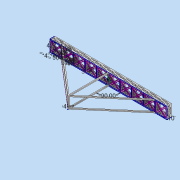
# Autodesk Inventor part: hashi1shado
Saved by Autodesk Inventor 2022 (Build 260153000, 153)
## iProperties
Created: 2024-05-14
Part Number: hashi1shado
Material: 一般
Document SubType Name: Modeling
Designer: ktamu
Density: 1 g/cm^3
Appearance: 既定
Mass: 137.691 g
Surface Area: 1271.48 cm^2
Volume: 137.691 cm^3
Author: ktamu
Autodesk Inventor part; units mm, degrees
ref_plane "YZ Plane" through (0, 0, 0) normal (1, 0, 0) x (0, 1, 0)
ref_plane "XZ Plane" through (0, 0, 0) normal (0, 1, 0) x (-1, 0, 0)
ref_plane "XY Plane" through (0, 0, 0) normal (0, 0, 1) x (1, 0, 0)
sketch "スケッチ2" plane through (0, 0, 0) normal (1, 0, 0) x (0, 1, 0)
  line L0 (25, 10) -> (-25, 10)
  line L1 (-25, 10) -> (-25, -10)
  line L2 (-25, -10) -> (25, -10)
  line L3 (25, -10) -> (25, 10)
  line L4 (25, 10) -> (-25, -10) construction
  line L5 (-25, 10) -> (25, -10) construction
  point P0 (0, 0)
  dimension "d4" = 50
  dimension "d5" = 20
  constraints: 12 end point, 2 midpoint, 2 parallel, 1 horizontal, 1 perpendicular
  measures "d4" distance of L2.end L1.end
  measures "d5" distance of L1.end L0.end
extrude "押し出し2" add sketch "スケッチ2" along normal mid plane 500
sketch "スケッチ3" plane through (-250, -25, 10) normal (0, 0, 1) x (1, 0, 0)
  circle A0 centre (250, 25) radius 5
  dimension "d8" = 10
  constraints: 1 centre point, 1 coincident
  measures "d8" diameter of A0
extrude "押し出し3" add sketch "スケッチ3" along normal blind 2
sketch "SCfront" plane through (-250, -25, 10) normal (0, -1, 0) x (1, 0, 0)
  line L0 (0, -20) -> (500, -20) projected
  line L1 (500, 0) -> (500, -20) projected
  line L2 (500, 0) -> (0, 0) projected
  line L3 (0, -20) -> (0, 0) projected
  line L4 (0, 0) -> (500, 0)
  line L5 (500, 0) -> (500, -20)
  line L6 (500, -20) -> (0, -20)
  line L7 (0, -20) -> (0, 0)
  line L8 (0, 0) -> (500, -20) construction
  line L9 (500, 0) -> (0, -20) construction
  line L10 (0, 0) -> (500, 0) projected
  line L11 (0, -20) -> (500, -20) projected
  line L12 (0, 0) -> (50, 0)
  line L13 (50, 0) -> (50, -20)
  line L14 (50, -20) -> (0, -20)
  line L15 (0, -20) -> (0, 0)
  line L16 (100, 0) -> (100, -20)
  line L17 (150, 0) -> (150, -20)
  line L18 (200, 0) -> (200, -20)
  line L19 (250, 0) -> (250, -20)
  line L20 (450, 0) -> (450, -20)
  line L21 (400, 0) -> (400, -20)
  line L22 (350, 0) -> (350, -20)
  line L23 (300, 0) -> (300, -20)
  line L24 (0, 0) -> (0, -20) projected
  line L25 (0, 0) -> (50, -20)
  line L26 (0, -20) -> (50, 0) construction
  line L27 (50, 0) -> (100, -20)
  line L28 (100, 0) -> (50, -20)
  line L29 (52, -4) -> (98, -4)
  line L30 (98, -4) -> (98, -16)
  line L31 (98, -16) -> (52, -16)
  line L32 (52, -16) -> (52, -4)
  line L33 (75, -10) -> (98, -16) construction
  line L34 (98, -4) -> (52, -16) construction
  line L35 (102, -4) -> (148, -4)
  line L36 (102, -16) -> (102, -4)
  line L37 (148, -16) -> (102, -16)
  line L38 (148, -4) -> (148, -16)
  line L39 (152, -4) -> (198, -4)
  line L40 (152, -16) -> (152, -4)
  line L41 (198, -16) -> (152, -16)
  line L42 (198, -4) -> (198, -16)
  line L43 (202, -4) -> (248, -4)
  line L44 (202, -16) -> (202, -4)
  line L45 (248, -16) -> (202, -16)
  line L46 (248, -4) -> (248, -16)
  line L47 (252, -4) -> (298, -4)
  line L48 (252, -16) -> (252, -4)
  line L49 (298, -16) -> (252, -16)
  line L50 (298, -4) -> (298, -16)
  line L51 (302, -4) -> (348, -4)
  line L52 (302, -16) -> (302, -4)
  line L53 (348, -16) -> (302, -16)
  line L54 (348, -4) -> (348, -16)
  line L55 (352, -4) -> (398, -4)
  line L56 (352, -16) -> (352, -4)
  line L57 (398, -16) -> (352, -16)
  line L58 (398, -4) -> (398, -16)
  line L59 (402, -4) -> (448, -4)
  line L60 (402, -16) -> (402, -4)
  line L61 (448, -16) -> (402, -16)
  line L62 (448, -4) -> (448, -16)
  line L63 (48, -4) -> (48, -16)
  line L64 (48, -4) -> (4, -4)
  line L65 (4, -4) -> (4, -16.3421)
  line L66 (4, -16.3421) -> (48, -16.3421)
  line L67 (48, -16.3421) -> (48, -4)
  line L68 (452, -4) -> (452, -16)
  line L69 (452, -4) -> (496, -4)
  line L70 (496, -4) -> (496, -16.3421)
  line L71 (496, -16.3421) -> (452, -16.3421)
  line L72 (11.4052, -4) -> (48, -14.2649)
  line L73 (4, -6.0772) -> (40.5948, -16.3421)
  line L74 (488.5948, -4) -> (452, -14.2649)
  line L75 (496, -6.0772) -> (459.4052, -16.3421)
  line L76 (52, -4) -> (75, -10)
  line L77 (52, -6.0669) -> (90.0768, -16)
  line L78 (52.5048, -2.0648) -> (52.6652, -2.1066)
  line L79 (59.9232, -4) -> (98, -13.9331)
  line L80 (109.9232, -4) -> (148, -13.9331)
  line L81 (102, -6.0669) -> (140.0768, -16)
  line L82 (159.9232, -4) -> (198, -13.9331)
  line L83 (152, -6.0669) -> (190.0768, -16)
  line L84 (209.9232, -4) -> (248, -13.9331)
  line L85 (202, -6.0669) -> (240.0768, -16)
  line L86 (448, -6.0669) -> (409.9232, -16)
  line L87 (440.0768, -4) -> (402, -13.9331)
  line L88 (390.0768, -4) -> (352, -13.9331)
  line L89 (398, -6.0669) -> (359.9232, -16)
  line L90 (340.0768, -4) -> (302, -13.9331)
  line L91 (348, -6.0669) -> (309.9232, -16)
  line L92 (290.0768, -4) -> (252, -13.9331)
  line L93 (298, -6.0669) -> (259.9232, -16)
  line L94 (0, -10) -> (496, -10) construction
  line L95 (0, -10) -> (496, -10) construction
  line L96 (11.4052, -16) -> (48, -5.7351)
  line L97 (4, -13.9228) -> (39.375, -4)
  line L98 (488.5948, -16) -> (452, -5.7351)
  line L99 (496, -13.9228) -> (459.4052, -3.6579)
  line L100 (52, -13.9331) -> (90.0768, -4)
  line L101 (59.9232, -16) -> (98, -6.0669)
  line L102 (109.9232, -16) -> (148, -6.0669)
  line L103 (102, -13.9331) -> (140.0768, -4)
  line L104 (159.9232, -16) -> (198, -6.0669)
  line L105 (152, -13.9331) -> (190.0768, -4)
  line L106 (209.9232, -16) -> (248, -6.0669)
  line L107 (202, -13.9331) -> (240.0768, -4)
  line L108 (448, -13.9331) -> (409.9232, -4)
  line L109 (440.0768, -16) -> (402, -6.0669)
  line L110 (398, -13.9331) -> (359.9232, -4)
  line L111 (390.0768, -16) -> (352, -6.0669)
  line L112 (348, -13.9331) -> (309.9232, -4)
  line L113 (340.0768, -16) -> (302, -6.0669)
  line L114 (298, -13.9331) -> (259.9232, -4)
  line L115 (290.0768, -16) -> (252, -6.0669)
  line L116 (25.3901, -12.0772) -> (10.1855, -16.3421)
  line L117 (474.6099, -12.0772) -> (489.8145, -16.3421)
  line L118 (150, 0) -> (313.5157, 0) construction
  line L119 (250, 0) -> (250, 173.2051)
  line L120 (250, 0) -> (423.2051, 0) construction
  line L121 (248, -20) -> (248, 0)
  line L122 (248, 0) -> (248, 166.2211)
  line L123 (152, -0.5359) -> (152, -20)
  line L124 (252, -20) -> (252, 0)
  line L125 (148, 0.5359) -> (148, -20)
  line L126 (250, 173.2051) -> (250, 177.2051)
  line L127 (150, 0) -> (152, 3.4641)
  line L128 (248, 166.2211) -> (54.1451, 0)
  line L129 (48, 0) -> (250, 173.2051)
  point P0 (250, -10)
  point P1 (440.0768, -4)
  point P2 (390.0768, -4)
  point P3 (340.0768, -4)
  point P4 (290.0768, -4)
  point P5 (209.9232, -4)
  point P6 (159.9232, -4)
  point P7 (109.9232, -4)
  point P8 (60.1439, -4.0576)
  point P9 (60, -4)
  point P10 (90, -16)
  point P11 (89.8561, -15.9424)
  point P12 (48, -14.2649)
  point P13 (40.5948, -3.6579)
  point P14 (482.0151, -10)
  point P15 (474.6099, -7.9228)
  point P16 (460.625, -4)
  point P17 (467.2046, -10)
  point P18 (432.9232, -10)
  point P19 (425, -12.0669)
  point P20 (425, -7.9331)
  point P21 (417.0768, -10)
  point P22 (382.9232, -10)
  point P23 (375, -12.0669)
  point P24 (375, -7.9331)
  point P25 (367.0768, -10)
  point P26 (332.9232, -10)
  point P27 (325, -12.0669)
  point P28 (325, -7.9331)
  point P29 (317.0768, -10)
  point P30 (282.9232, -10)
  point P31 (275, -12.0669)
  point P32 (275, -7.9331)
  point P33 (267.0768, -10)
  point P34 (232.9232, -10)
  point P35 (225, -7.9331)
  point P36 (225, -12.0669)
  point P37 (217.0768, -10)
  point P38 (182.9232, -10)
  point P39 (175, -7.9331)
  point P40 (175, -12.0669)
  point P41 (167.0768, -10)
  point P42 (132.9232, -10)
  point P43 (125, -7.9331)
  point P44 (125, -12.0669)
  point P45 (117.0768, -10)
  point P46 (67.0768, -10)
  point P47 (59.9232, -16)
  point P48 (75, -12.0669)
  point P49 (75, -7.9331)
  point P50 (82.9232, -10)
  point P51 (25.3901, -7.9228)
  point P52 (32.7954, -10)
  point P53 (48, -5.7351)
  point P54 (11.4052, -16)
  point P55 (17.9849, -10)
  point P56 (4, -13.9228)
  point P57 (148, 0)
  point P58 (54.1451, 0)
  point P59 (48, 0)
  dimension "d12" = 50
  dimension "d15" = 50
  dimension "d20" = 46
  dimension "d21" = 12
  dimension "d24" = 50
  dimension "d29" = 4
  dimension "d30" = 4
  dimension "d33" = 4
  dimension "d37" = 2
  dimension "d40" = 50
  dimension "d96" = 0
  dimension "d97" = 10
  dimension "d105" = 90
  dimension "d116" = 4
  constraints: 246 end point, 73 symmetric about line, 25 point on line, 12 parallel, 10 horizontal, 6 midpoint, 4 perpendicular, 2 equal length, 1 vertical, 87 other
  measures "d12" distance of L13.end L14.end
  measures "d15" distance of L12.end L16.start
  measures "d20" distance of L30.end L31.end
  measures "d21" distance of L29.end L30.end
  measures "d24" distance of L29.start L35.start
  measures "d29" distance between parallel lines of L32 L63
  measures "d30" distance between parallel lines of L65 L3
  measures "d33" distance between parallel lines of L12 L64
  measures "d37" distance between parallel lines of L76 L77
  measures "d40" distance of L79.start L80.start
  measures "d96" distance between parallel lines of L94 L95
  measures "d97" distance between parallel lines of L0 L95
  measures "d105" angle of L120 L119
  measures "d116" distance between parallel lines of L129 L128
extrude "押し出し4" cut sketch "SCfront" against normal through all contours L31 L101 L28 | L28 L101 L77 L27 L31 | L29 L28 L100 L79 L27 | L66 L116 L96 L73 | L101 L31 L32 L100 L77 L28 | L28 L77 L101 | L64 L97 L72 | L29 L100 L28 | L96 L116 L66 L65 L97 L73 | L96 L63 L72 | L72 L97 L64 L63 L96 | L97 L65 L73 | L37 L102 L81 | L80 L102 L38 | L38 L102 L80 L103 L35 | L100 L29 L30 L101 L79 L28 | L28 L79 L100 | L100 L32 L77 | L37 L36 L103 L81 L102 | L103 L80 L35 | L101 L30 L79 | L46 L106 L84 L107 L43 | L47 L114 L92 L115 L48 | L103 L36 L81 | L107 L84 L43 | L46 L84 L106 | L47 L92 L114 | L115 L92 L48 | L45 L106 L85 | L93 L115 L49 | L107 L44 L85 | L85 L106 L45 L44 L107 | L114 L50 L49 L115 L93 | L93 L50 L114 | L39 L105 L82 | L83 L105 L40 | L39 L42 L104 L82 L105 | L105 L83 L104 L41 L40 | L104 L42 L82 | L83 L41 L104 | L51 L112 L90 L113 L52 | L51 L90 L112 | L113 L90 L52 | L112 L54 L53 L113 L91 | L91 L54 L112 | L113 L53 L91 | L55 L110 L88 L111 L56 | L55 L88 L110 | L111 L88 L56 | L110 L58 L57 L111 L89 | L89 L58 L110 | L111 L57 L89 | L59 L108 L87 L109 L60 | L59 L87 L108 | L109 L87 L60 | L108 L62 L61 L109 L86 | L86 L62 L108 | L109 L61 L86 | L69 L99 L74 L98 L68 | L98 L74 L68 | L69 L74 L99 | L98 L117 L71 L75 | L75 L99 L70 L71 L117 L98 | L75 L70 L99
sketch "SCLeft" plane through (-250, 0, 0) normal (-1, 0, 0) x (0, 0, 1)
  line L0 (10, 25) -> (10, -25) projected
  line L1 (-10, 25) -> (10, 25)
  line L2 (10, 25) -> (10, -25)
  line L3 (10, -25) -> (-10, -25)
  line L4 (-10, -25) -> (-10, 25)
  line L5 (-10, 25) -> (10, -25) construction
  line L6 (10, 25) -> (-10, -25) construction
  line L7 (-6, 21) -> (6, 21)
  line L8 (6, 21) -> (6, -21)
  line L9 (6, -21) -> (-6, -21)
  line L10 (-6, -21) -> (-6, 21)
  line L11 (-6, 21) -> (-1.04, 3.6401) construction
  line L12 (6, 21) -> (-6, -21) construction
  line L13 (7.4154, 0) -> (4.3427, 0)
  line L14 (2.08, 0) -> (6, -13.7199)
  line L15 (-3.92, 21) -> (0, 7.2801)
  line L16 (-6, 21) -> (-1.04, 3.6401)
  line L17 (1.04, -3.6401) -> (6, -21)
  line L18 (-6, 13.7199) -> (-2.08, 0)
  line L19 (0, -7.2801) -> (3.92, -21)
  line L20 (0, 7.2801) -> (3.92, 21)
  line L21 (-6, -13.7199) -> (-2.08, 0)
  line L22 (-3.92, -21) -> (0, -7.2801)
  line L23 (2.08, 0) -> (6, 13.7199)
  point P0 (0, 0)
  dimension "d47" = 12
  dimension "d48" = 42
  constraints: 46 end point, 8 parallel, 5 point on line, 4 symmetric about line, 3 horizontal, 3 midpoint, 2 perpendicular
  measures "d47" distance of L8.end L9.end
  measures "d48" distance of L7.end L8.end
extrude "押し出し5left" cut sketch "SCLeft" against normal through all contours L7 L15 L20 L8 L23 L14 L9 L19 L22 L10 L21 L18 | L7 L20 L15 | L18 L21 L10 | L8 L14 L23 | L22 L19 L9
extrude "押し出し6" add sketch "SCLeft" against normal blind 4 contours L7 L15 L20 L8 L23 L14 L9 L19 L22 L10 L21 L18
mirror "ミラー1" about plane through (0, 0, 0) normal (1, 0, 0) of "押し出し6"
sketch "SCtop" plane through (-250, -25, 10) normal (0, 0, 1) x (1, 0, 0)
  circle A0 centre (250, 25) radius 5 projected
  line L0 (500, 0) -> (0, 0) projected
  line L1 (500, 50) -> (500, 0) projected
  line L2 (0, 50) -> (500, 50) projected
  line L3 (0, 0) -> (0, 50) projected
  circle A1 centre (250, 25) radius 5 projected
  line L4 (0, 0) -> (0, 50) projected
  line L5 (0, 50) -> (500, 0) construction
  line L6 (0, 0) -> (500, 0) projected
  line L7 (500, 50) -> (0, 0) construction
  line L8 (0, 50) -> (500, 50)
  line L9 (500, 50) -> (500, 0)
  line L10 (500, 0) -> (0, 0)
  line L11 (0, 0) -> (0, 50)
  line L12 (0, 50) -> (500, 0) construction
  line L13 (500, 50) -> (0, 0) construction
  line L14 (0, 50) -> (500, 50) projected
  line L15 (0, 50) -> (50, 50)
  line L16 (50, 50) -> (50, 0)
  line L17 (50, 0) -> (0, 0)
  line L18 (0, 0) -> (0, 50)
  line L19 (100, 50) -> (100, 0)
  line L20 (150, 50) -> (150, 0)
  line L21 (200, 50) -> (200, 0)
  line L22 (250, 50) -> (250, 0)
  line L23 (300, 50) -> (300, 0)
  line L24 (350, 50) -> (350, 0)
  line L25 (400, 50) -> (400, 0)
  line L26 (450, 50) -> (450, 0)
  line L27 (50, 50) -> (100, 0)
  line L28 (0, 50) -> (50, 0)
  line L29 (50, 50) -> (0, 0)
  line L30 (98, 4) -> (60.1439, 4) projected
  line L31 (52, 46) -> (98, 46)
  line L32 (98, 46) -> (98, 4)
  line L33 (98, 4) -> (52, 4)
  line L34 (52, 4) -> (52, 46)
  line L35 (4, 46) -> (48, 46)
  line L36 (48, 46) -> (48, 4)
  line L37 (48, 4) -> (4, 4)
  line L38 (4, 4) -> (4, 46)
  line L39 (6.8284, 46) -> (48.0258, 4.8026)
  line L40 (4, 43.1716) -> (43.1716, 4)
  line L41 (25, 25) -> (25, 18.6219)
  line L42 (98, 0) -> (98, 4) projected
  line L43 (53.4759, 44.6524) -> (98, 4)
  line L44 (52, 43.2918) -> (95.0338, 4)
  line L45 (54.9662, 46) -> (98, 6.7082)
  line L46 (98, 43.2918) -> (54.9662, 4)
  line L47 (92.2747, 40.7725) -> (53.4759, 5.3476)
  line L48 (95.0338, 46) -> (52, 6.7082)
  line L49 (50.1449, 5.0145) -> (50, 4.8822)
  line L50 (73.5843, 23.5843) -> (90.9091, 40.9091)
  line L51 (92.2747, 40.7725) -> (73.5169, 23.6459) construction
  line L52 (53.4759, 5.3476) -> (52, 4) construction
  line L53 (52, 46) -> (53.4759, 44.6524) construction
  line L54 (73.5169, 26.3541) -> (98, 4) construction
  line L55 (48, 46) -> (4, 4)
  line L56 (45.1034, 46) -> (4, 6.7649)
  line L57 (48, 43.2351) -> (6.8966, 4)
  line L58 (104.9662, 46) -> (148, 6.7082)
  line L59 (145.0338, 46) -> (102, 6.7082)
  line L60 (148, 43.2918) -> (104.9662, 4)
  line L61 (102, 43.2918) -> (145.0338, 4)
  line L62 (148, 46) -> (148, 4)
  line L63 (102, 46) -> (148, 46)
  line L64 (102, 4) -> (102, 46)
  line L65 (148, 4) -> (102, 4)
  line L66 (154.9662, 46) -> (198, 6.7082)
  line L67 (195.0338, 46) -> (152, 6.7082)
  line L68 (198, 43.2918) -> (154.9662, 4)
  line L69 (152, 43.2918) -> (195.0338, 4)
  line L70 (198, 46) -> (198, 4)
  line L71 (152, 46) -> (198, 46)
  line L72 (152, 4) -> (152, 46)
  line L73 (198, 4) -> (152, 4)
  line L74 (204.9662, 46) -> (248, 6.7082)
  line L75 (245.0338, 46) -> (202, 6.7082)
  line L76 (248, 43.2918) -> (204.9662, 4)
  line L77 (202, 43.2918) -> (245.0338, 4)
  line L78 (248, 46) -> (248, 4)
  line L79 (202, 46) -> (248, 46)
  line L80 (202, 4) -> (202, 46)
  line L81 (248, 4) -> (202, 4)
  line L82 (254.9662, 46) -> (298, 6.7082)
  line L83 (295.0338, 46) -> (252, 6.7082)
  line L84 (298, 43.2918) -> (254.9662, 4)
  line L85 (252, 43.2918) -> (295.0338, 4)
  line L86 (298, 46) -> (298, 4)
  line L87 (252, 46) -> (298, 46)
  line L88 (252, 4) -> (252, 46)
  line L89 (298, 4) -> (252, 4)
  line L90 (304.9662, 46) -> (348, 6.7082)
  line L91 (345.0338, 46) -> (302, 6.7082)
  line L92 (348, 43.2918) -> (304.9662, 4)
  line L93 (302, 43.2918) -> (345.0338, 4)
  line L94 (348, 46) -> (348, 4)
  line L95 (302, 46) -> (348, 46)
  line L96 (302, 4) -> (302, 46)
  line L97 (348, 4) -> (302, 4)
  line L98 (354.9662, 46) -> (398, 6.7082)
  line L99 (395.0338, 46) -> (352, 6.7082)
  line L100 (398, 43.2918) -> (354.9662, 4)
  line L101 (352, 43.2918) -> (395.0338, 4)
  line L102 (398, 46) -> (398, 4)
  line L103 (352, 46) -> (398, 46)
  line L104 (352, 4) -> (352, 46)
  line L105 (398, 4) -> (352, 4)
  line L106 (404.9662, 46) -> (448, 6.7082)
  line L107 (445.0338, 46) -> (402, 6.7082)
  line L108 (448, 43.2918) -> (404.9662, 4)
  line L109 (402, 43.2918) -> (445.0338, 4)
  line L110 (448, 46) -> (448, 4)
  line L111 (402, 46) -> (448, 46)
  line L112 (402, 4) -> (402, 46)
  line L113 (448, 4) -> (402, 4)
  line L114 (496, 46) -> (452, 46)
  line L115 (452, 46) -> (452, 4)
  line L116 (452, 4) -> (496, 4)
  line L117 (496, 4) -> (496, 46)
  line L118 (493.1716, 46) -> (451.9742, 4.8026)
  line L119 (496, 43.1716) -> (456.8284, 4)
  line L120 (454.8966, 46) -> (496, 6.7649)
  line L121 (452, 43.2351) -> (493.1034, 4)
  point P0 (75, 25)
  point P1 (123.5169, 26.3541)
  point P2 (123.5843, 23.5843)
  point P3 (123.5169, 23.6459)
  point P4 (173.5169, 26.3541)
  point P5 (173.5843, 23.5843)
  point P6 (173.5169, 23.6459)
  point P7 (223.5169, 26.3541)
  point P8 (223.5843, 23.5843)
  point P9 (223.5169, 23.6459)
  point P10 (273.5169, 26.3541)
  point P11 (273.5843, 23.5843)
  point P12 (273.5169, 23.6459)
  point P13 (323.5169, 26.3541)
  point P14 (323.5843, 23.5843)
  point P15 (323.5169, 23.6459)
  point P16 (373.5169, 26.3541)
  point P17 (373.5843, 23.5843)
  point P18 (373.5169, 23.6459)
  point P19 (423.5169, 26.3541)
  point P20 (423.5843, 23.5843)
  point P21 (423.5169, 23.6459)
  point P22 (474.5441, 21.7157)
  point P23 (477.3733, 24.5449)
  point P24 (474.4791, 27.3075)
  point P25 (452, 4.8284)
  point P26 (471.6499, 24.4784)
  point P27 (427.9662, 25)
  point P28 (425, 22.2918)
  point P29 (425, 27.7082)
  point P30 (375, 22.2918)
  point P31 (375, 27.7082)
  point P32 (422.0338, 25)
  point P33 (377.9662, 25)
  point P34 (372.0338, 25)
  point P35 (327.9662, 25)
  point P36 (325, 22.2918)
  point P37 (325, 27.7082)
  point P38 (322.0338, 25)
  point P39 (275, 22.2918)
  point P40 (277.9662, 25)
  point P41 (275, 27.7082)
  point P42 (252, 20.4174)
  point P43 (272.0338, 25)
  point P44 (252, 29.5826)
  point P45 (225, 22.2918)
  point P46 (248, 29.5826)
  point P47 (227.9662, 25)
  point P48 (248, 20.4174)
  point P49 (225, 27.7082)
  point P50 (222.0338, 25)
  point P51 (175, 22.2918)
  point P52 (177.9662, 25)
  point P53 (175, 27.7082)
  point P54 (172.0338, 25)
  point P55 (125, 22.2918)
  point P56 (127.9662, 25)
  point P57 (125, 27.7082)
  point P58 (122.0338, 25)
  point P59 (77.9662, 25)
  point P60 (75, 22.2918)
  point P61 (75, 27.7082)
  point P62 (72.0338, 25)
  point P63 (25.4559, 21.7157)
  point P64 (28.3501, 24.4784)
  point P65 (48, 4.8284)
  point P66 (22.6267, 24.5449)
  point P67 (25.5209, 27.3075)
  dimension "d55" = 50
  dimension "d56" = 50
  dimension "d59" = 50
  dimension "d64" = 46
  dimension "d65" = 42
  dimension "d66" = 44
  dimension "d67" = 42
  dimension "d68" = 4
  dimension "d69" = 4
  dimension "d76" = 2
  dimension "d77" = 2
  dimension "d80" = 50
  constraints: 226 end point, 97 point on line, 20 midpoint, 17 parallel, 12 symmetric about line, 6 horizontal, 5 perpendicular, 1 vertical, 185 other
  measures "d55" distance of L16.end L17.end
  measures "d56" distance of L15.end L16.end
  measures "d59" distance of L15.end L19.start
  measures "d64" distance of L30.start L33.end
  measures "d65" distance of L31.end L30.start
  measures "d66" distance of L36.end L37.end
  measures "d67" distance of L35.end L36.end
  measures "d68" distance between parallel lines of L2 L35
  measures "d69" distance between parallel lines of L34 L36
  measures "d76" distance between parallel lines of L55 L56
  measures "d77" distance between parallel lines of L55 L57
  measures "d80" distance of L45.start L58.start
extrude "押し出し7" cut sketch "SCtop" against normal through all contours A0 L88 L85 L83 | A0 L78 L74 L76 | L82 L87 L83 | L85 L89 L84 | L84 L86 L82 | L74 L79 L75 | L77 L81 L76 | L75 L80 L77 | L31 L48 L45 | L56 L39 L35 | L30 L33 L46 L44 | L45 L46 L32 | L40 L56 L38 | L44 L48 L34 | L36 L39 L57 | L37 L57 L40 | L63 L59 L58 | L60 L62 L58 | L59 L64 L61 | L61 L65 L60 | L71 L67 L66 | L68 L70 L66 | L67 L72 L69 | L69 L73 L68 | L95 L91 L90 | L92 L94 L90 | L91 L96 L93 | L93 L97 L92 | L103 L99 L98 | L100 L102 L98 | L99 L104 L101 | L101 L105 L100 | L111 L107 L106 | L108 L110 L106 | L107 L112 L109 | L109 L113 L108 | L118 L120 L114 | L117 L120 L119 | L118 L115 L121 | L121 L116 L119
sketch "スケッチ7" plane through (0, 0, 12) normal (0, 0, 1) x (1, 0, 0)
  line L0 (-2, 21) -> (-2, -21) projected
  line L1 (2, -18.2918) -> (2, -4.5826) projected
  line L2 (2, -21) -> (2, 21) projected
  circle A0 centre (0, 0) radius 5 projected
  arc A1 (-2, -4.5826) -> (2, -4.5826) centre (0, 0) ccw projected
  line L3 (-2, -4.5826) -> (-2, 4.5826)
  line L4 (2, -4.5826) -> (2, 4.5826)
  circle A2 centre (0, 0) radius 1
  point P0 (-2, -4.5826)
  dimension "d89" = 2
  constraints: 4 end point, 2 point on circle, 2 point on line, 1 centre point, 1 coincident
  measures "d89" diameter of A2
extrude "押し出し8" cut sketch "スケッチ7" against normal through all contours L0 A0 | A0 L2
extrude "押し出し9" cut sketch "スケッチ7" against normal blind 2 contours A0 L2 L0
extrude "押し出し10" cut sketch "スケッチ7" against normal blind 1 contours A2
extrude "押し出し11" cut sketch "スケッチ7" against normal blind 2 contours A2
extrude "押し出し12" add sketch "SCfront" against normal blind 4 contours L101 L31 L32 L100 L77 L28 | L28 L77 L101 | L96 L116 L66 L65 L97 L73 | L72 L97 L64 L63 L96 | L38 L102 L80 L103 L35 | L100 L29 L30 L101 L79 L28 | L28 L79 L100 | L37 L36 L103 L81 L102 | L46 L106 L84 L107 L43 | L47 L114 L92 L115 L48 | L85 L106 L45 L44 L107 | L114 L50 L49 L115 L93 | L39 L42 L104 L82 L105 | L105 L83 L104 L41 L40 | L51 L112 L90 L113 L52 | L112 L54 L53 L113 L91 | L55 L110 L88 L111 L56 | L110 L58 L57 L111 L89 | L59 L108 L87 L109 L60 | L108 L62 L61 L109 L86 | L69 L99 L74 L98 L68 | L98 L117 L71 L75 | L75 L99 L70 L71 L117 L98
extrude "押し出し13" cut sketch "SCfront" against normal blind 88.5 contours L98 L117 L71 L75
mirror "ミラー2" about plane through (0, 0, 0) normal (0, 1, 0) of "押し出し12"
extrude "押し出し14" cut sketch "SCfront" against normal blind 84 contours L98 L117 L71 L75
extrude "押し出し15" add sketch "SCfront" against normal blind 4 contours L2 L128 L122
mirror "ミラー3" about plane through (0, 0, 0) normal (1, 0, 0) of "押し出し15"
mirror "ミラー4" about plane through (0, 0, 0) normal (0, 1, 0) of "押し出し15", "ミラー3"
extrude "押し出し16" cut sketch "SCfront" against normal through all contours L2 L128 L122
sketch "スケッチ10" plane through (-250, -25, -10) normal (0, -1, 0) x (1, 0, 0)
  line L0 (252, 20) -> (0, 20) projected
  line L1 (0, 0) -> (0, 20) projected
  line L2 (0, 0) -> (500, 0) projected
  line L3 (500, 20) -> (500, 0) projected
  line L4 (500, 20) -> (445.8549, 20) projected
  line L5 (252, 186.2211) -> (445.8549, 20) projected
  line L6 (252, 20) -> (252, 186.2211) projected
  line L7 (459.4052, 3.6579) -> (474.6099, 7.9228) projected
  line L8 (474.6099, 7.9228) -> (489.8145, 3.6579) projected
  line L9 (489.8145, 3.6579) -> (459.4052, 3.6579) projected
  line L10 (98, 13.9331) -> (98, 6.0669) projected
  line L11 (98, 6.0669) -> (82.9232, 10) projected
  line L12 (82.9232, 10) -> (98, 13.9331) projected
  line L13 (152, 6.0669) -> (152, 13.9331) projected
  line L14 (152, 13.9331) -> (167.0768, 10) projected
  line L15 (167.0768, 10) -> (152, 6.0669) projected
  line L16 (267.0768, 10) -> (252, 6.0669) projected
  line L17 (252, 6.0669) -> (252, 13.9331) projected
  line L18 (252, 13.9331) -> (267.0768, 10) projected
  line L19 (367.0768, 10) -> (352, 6.0669) projected
  line L20 (352, 6.0669) -> (352, 13.9331) projected
  line L21 (352, 13.9331) -> (367.0768, 10) projected
  line L22 (467.2046, 10) -> (452, 5.7351) projected
  line L23 (452, 5.7351) -> (452, 14.2649) projected
  line L24 (452, 14.2649) -> (467.2046, 10) projected
  line L25 (440.0768, 4) -> (409.9232, 4) projected
  line L26 (409.9232, 4) -> (425, 7.9331) projected
  line L27 (425, 7.9331) -> (440.0768, 4) projected
  line L28 (340.0768, 4) -> (309.9232, 4) projected
  line L29 (309.9232, 4) -> (325, 7.9331) projected
  line L30 (325, 7.9331) -> (340.0768, 4) projected
  line L31 (225, 12.0669) -> (209.9232, 16) projected
  line L32 (209.9232, 16) -> (240.0768, 16) projected
  line L33 (240.0768, 16) -> (225, 12.0669) projected
  line L34 (125, 12.0669) -> (109.9232, 16) projected
  line L35 (109.9232, 16) -> (140.0768, 16) projected
  line L36 (140.0768, 16) -> (125, 12.0669) projected
  line L37 (48, 14.2649) -> (48, 5.7351) projected
  line L38 (48, 5.7351) -> (32.7954, 10) projected
  line L39 (32.7954, 10) -> (48, 14.2649) projected
  line L40 (75, 7.9331) -> (89.8561, 4.0576) projected
  line L41 (89.8561, 4.0576) -> (90, 4) projected
  line L42 (90, 4) -> (59.9232, 4) projected
  line L43 (59.9232, 4) -> (75, 7.9331) projected
  line L44 (175, 12.0669) -> (159.9232, 16) projected
  line L45 (159.9232, 16) -> (190.0768, 16) projected
  line L46 (190.0768, 16) -> (175, 12.0669) projected
  line L47 (290.0768, 4) -> (259.9232, 4) projected
  line L48 (259.9232, 4) -> (275, 7.9331) projected
  line L49 (275, 7.9331) -> (290.0768, 4) projected
  line L50 (390.0768, 4) -> (359.9232, 4) projected
  line L51 (359.9232, 4) -> (375, 7.9331) projected
  line L52 (375, 7.9331) -> (390.0768, 4) projected
  line L53 (417.0768, 10) -> (402, 6.0669) projected
  line L54 (402, 6.0669) -> (402, 13.9331) projected
  line L55 (402, 13.9331) -> (417.0768, 10) projected
  line L56 (317.0768, 10) -> (302, 6.0669) projected
  line L57 (302, 6.0669) -> (302, 13.9331) projected
  line L58 (302, 13.9331) -> (317.0768, 10) projected
  line L59 (202, 6.0669) -> (202, 13.9331) projected
  line L60 (202, 13.9331) -> (217.0768, 10) projected
  line L61 (217.0768, 10) -> (202, 6.0669) projected
  line L62 (102, 6.0669) -> (102, 13.9331) projected
  line L63 (102, 13.9331) -> (117.0768, 10) projected
  line L64 (117.0768, 10) -> (102, 6.0669) projected
  line L65 (25.3901, 7.9228) -> (40.5948, 3.6579) projected
  line L66 (40.5948, 3.6579) -> (10.1855, 3.6579) projected
  line L67 (10.1855, 3.6579) -> (25.3901, 7.9228) projected
  line L68 (67.0768, 10) -> (52, 6.0669) projected
  line L69 (52, 6.0669) -> (52, 13.9331) projected
  line L70 (52, 13.9331) -> (67.0768, 10) projected
  line L71 (159.9232, 4) -> (175, 7.9331) projected
  line L72 (175, 7.9331) -> (190.0768, 4) projected
  line L73 (190.0768, 4) -> (159.9232, 4) projected
  line L74 (275, 12.0669) -> (259.9232, 16) projected
  line L75 (259.9232, 16) -> (290.0768, 16) projected
  line L76 (290.0768, 16) -> (275, 12.0669) projected
  line L77 (375, 12.0669) -> (359.9232, 16) projected
  line L78 (359.9232, 16) -> (390.0768, 16) projected
  line L79 (390.0768, 16) -> (375, 12.0669) projected
  line L80 (474.6099, 12.0772) -> (460.625, 16) projected
  line L81 (460.625, 16) -> (488.5948, 16) projected
  line L82 (488.5948, 16) -> (474.6099, 12.0772) projected
  line L83 (448, 6.0669) -> (432.9232, 10) projected
  line L84 (432.9232, 10) -> (448, 13.9331) projected
  line L85 (448, 13.9331) -> (448, 6.0669) projected
  line L86 (348, 6.0669) -> (332.9232, 10) projected
  line L87 (332.9232, 10) -> (348, 13.9331) projected
  line L88 (348, 13.9331) -> (348, 6.0669) projected
  line L89 (232.9232, 10) -> (248, 13.9331) projected
  line L90 (248, 13.9331) -> (248, 6.0669) projected
  line L91 (248, 6.0669) -> (232.9232, 10) projected
  line L92 (132.9232, 10) -> (148, 13.9331) projected
  line L93 (148, 13.9331) -> (148, 6.0669) projected
  line L94 (148, 6.0669) -> (132.9232, 10) projected
  line L95 (39.375, 16) -> (25.3901, 12.0772) projected
  line L96 (25.3901, 12.0772) -> (11.4052, 16) projected
  line L97 (11.4052, 16) -> (39.375, 16) projected
  line L98 (90.0768, 16) -> (75, 12.0669) projected
  line L99 (75, 12.0669) -> (60.1439, 15.9424) projected
  line L100 (60.1439, 15.9424) -> (60, 16) projected
  line L101 (60, 16) -> (90.0768, 16) projected
  line L102 (182.9232, 10) -> (198, 13.9331) projected
  line L103 (198, 13.9331) -> (198, 6.0669) projected
  line L104 (198, 6.0669) -> (182.9232, 10) projected
  line L105 (298, 6.0669) -> (282.9232, 10) projected
  line L106 (282.9232, 10) -> (298, 13.9331) projected
  line L107 (298, 13.9331) -> (298, 6.0669) projected
  line L108 (398, 6.0669) -> (382.9232, 10) projected
  line L109 (382.9232, 10) -> (398, 13.9331) projected
  line L110 (398, 13.9331) -> (398, 6.0669) projected
  line L111 (496, 13.9228) -> (496, 6.0772) projected
  line L112 (496, 6.0772) -> (482.0151, 10) projected
  line L113 (482.0151, 10) -> (496, 13.9228) projected
  line L114 (425, 12.0669) -> (409.9232, 16) projected
  line L115 (409.9232, 16) -> (440.0768, 16) projected
  line L116 (440.0768, 16) -> (425, 12.0669) projected
  line L117 (325, 12.0669) -> (309.9232, 16) projected
  line L118 (309.9232, 16) -> (340.0768, 16) projected
  line L119 (340.0768, 16) -> (325, 12.0669) projected
  line L120 (209.9232, 4) -> (225, 7.9331) projected
  line L121 (225, 7.9331) -> (240.0768, 4) projected
  line L122 (240.0768, 4) -> (209.9232, 4) projected
  line L123 (109.9232, 4) -> (125, 7.9331) projected
  line L124 (125, 7.9331) -> (140.0768, 4) projected
  line L125 (140.0768, 4) -> (109.9232, 4) projected
  line L126 (17.9849, 10) -> (4, 6.0772) projected
  line L127 (4, 6.0772) -> (4, 13.9228) projected
  line L128 (4, 13.9228) -> (17.9849, 10) projected
  line L129 (445.8549, 20) -> (252, 186.2211) projected
  line L130 (252, 20) -> (445.8549, 20)
  point P0 (250, 10)
  constraints: 2 end point, 1 horizontal
extrude "押し出し19" cut sketch "スケッチ10" against normal through all contours L6 L5 L130
extrude "押し出し20" add sketch "SCfront" against normal blind 4 contours L2 L129 L119 L122 L128
mirror "ミラー5" about plane through (0, 0, 0) normal (0, 1, 0) of "押し出し20"
mirror "ミラー6" about plane through (0, 0, 0) normal (1, 0, 0) of "押し出し20", "ミラー5"
sketch "スケッチ11" plane through (-2, 21, 10) normal (0, -1, 0) x (1, 0, 0)
  line L0 (0, 171.3236) -> (4, 171.3236)
  line L1 (4, 171.3236) -> (4, 167.3236)
  line L2 (4, 167.3236) -> (0, 167.3236)
  line L3 (0, 167.3236) -> (0, 171.3236)
  line L4 (-193.8549, 0) -> (-200, 0) projected
  line L5 (0, 166.2211) -> (-193.8549, 0) projected
  line L6 (0, 0) -> (0, 166.2211) projected
  line L7 (4, 0) -> (0, 0) projected
  line L8 (4, 0) -> (4, 166.2211) projected
  line L9 (4, 166.2211) -> (197.8549, 0) projected
  line L10 (204, 0) -> (197.8549, 0) projected
  line L11 (204, 0) -> (2, 173.2051) projected
  line L12 (-200, 0) -> (2, 173.2051) projected
  point P0 (2, -10)
  dimension "d121" = 4
  dimension "d122" = 4
  constraints: 8 end point, 2 parallel, 1 horizontal, 1 perpendicular
  measures "d121" distance of L1.end L2.end
  measures "d122" distance of L0.end L1.end
extrude "押し出し21" add sketch "スケッチ11" along normal blind 43.5 contours L0 L1 L2 L3
